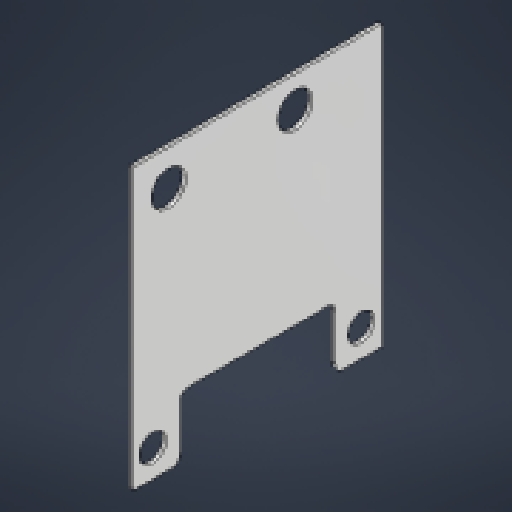
# Autodesk Inventor part: PLATE,FRONT
Saved by Autodesk Inventor 2026.1 (Build 301233020, 233B)
## iProperties
Created: 2026-03-30
Part Number: PLATE,FRONT
Material: Aluminum 6061-AHC
Document SubType Name: Sheet Metal
Designer: Owen L
Density: 2.7 g/cm^3
Sheet Metal Rule: Default
Appearance: Aluminum - Dark
Author: Owen L
Autodesk Inventor part; units mm, degrees
ref_plane "YZ Plane" through (0, 0, 0) normal (1, 0, 0) x (0, 1, 0)
ref_plane "XZ Plane" through (0, 0, 0) normal (0, 1, 0) x (-1, 0, 0)
ref_plane "XY Plane" through (0, 0, 0) normal (0, 0, 1) x (1, 0, 0)
sketch "Sketch1" plane through (0, 0, 0) normal (1, 0, 0) x (0, 1, 0)
  line L0 (-114.3, 101.6) -> (114.3, 101.6)
  line L1 (114.3, 101.6) -> (114.3, -101.6)
  line L2 (114.3, -101.6) -> (-114.3, -101.6)
  line L3 (-114.3, -101.6) -> (-114.3, 101.6)
  line L4 (-114.3, 101.6) -> (114.3, -101.6) construction
  line L5 (114.3, 101.6) -> (-114.3, -101.6) construction
  point P0 (0, 0)
  dimension "d0" = 228.6
  dimension "d1" = 203.2
  measures "d0" distance of L1.end L2.end
  measures "d1" distance of L0.end L1.end
extrude "Plate1" add sketch "Sketch1" along normal blind 3.175
sketch "Sketch2" plane through (3.175, 0, 0) normal (1, 0, 0) x (0, 0, -1)
  line L0 (-101.6, -114.3) -> (-101.6, 114.3) projected
  line L1 (-101.6, 114.3) -> (101.6, 114.3) projected
  circle A0 centre (-73.025, 85.217) radius 11.1125
  circle A1 centre (-85.725, -94.488) radius 11.1125
  circle A2 centre (84.455, -94.488) radius 11.1125
  line L2 (101.6, 114.3) -> (101.6, -114.3) projected
  circle A3 centre (30.3984, 88.9) radius 11.1125
  point P0 (0, 0)
  dimension "d3" = 28.575
  dimension "d4" = 29.083
  dimension "d5" = 22.225
  dimension "d9" = 15.875
  dimension "d11" = 22.225
  dimension "d19" = 103.489
  dimension "d20" = 25.4
  dimension "d21" = 170.18
  dimension "d23" = 208.788
  constraints: 4 centre point, 2 equal radius, 1 coincident, 1 horizontal alignment
  measures "d3" distance from line of L0 point (-73.025, 85.217)
  measures "d4" distance from line of L1 point (-73.025, 85.217)
  measures "d5" diameter of A0
  measures "d9" distance from line of L0 A1.centre
  measures "d11" diameter of A1
  measures "d19" distance of point (-73.025, 85.217) A3.centre
  measures "d20" distance from line of L1 A3.centre
  measures "d21" distance of A1.centre A2.centre
  measures "d23" distance from line of A1.centre L1
extrude "Cut1" cut sketch "Sketch2" against normal blind 3.175
sketch "Sketch3" plane through (3.175, 0, 0) normal (1, 0, 0) x (0, 0, -1)
  line L0 (-101.6, -114.3) -> (101.6, -114.3) projected
  line L1 (-63.5, -114.3) -> (63.5, -114.3)
  line L2 (63.5, -114.3) -> (63.5, -63.5)
  line L3 (63.5, -63.5) -> (-63.5, -63.5)
  line L4 (-63.5, -63.5) -> (-63.5, -114.3)
  point P0 (0, 0)
  point P1 (0, -63.5)
  point P2 (0, -114.3)
  dimension "d12" = 127
  dimension "d13" = 50.8
  constraints: 8 end point, 2 midpoint, 2 parallel, 1 horizontal, 1 perpendicular, 1 point on line, 1 vertical alignment
  measures "d12" distance of L3.end L2.end
  measures "d13" distance of L3.end L1.start
extrude "Cut2" cut sketch "Sketch3" against normal blind 3.175
fillet "Corner Round1" radius 6.35 4 edges at (1.5875, -114.3, 63.5) (1.5875, -63.5, 63.5) (1.5875, -114.3, -63.5) (1.5875, -63.5, -63.5)
equation "\"d6\" = Thickness"
equation "\"d14\" = Thickness"
equation "\"d2\" = Thickness"
equation "\"BendRadius\" = Thickness"
equation "\"BendReliefWidth\" = Thickness"
equation "\"BendReliefDepth\" = 0.5 * Thickness"
equation "\"CornerReliefSize\" = 4 * Thickness"
equation "\"MinimumRemnant\" = 2 * Thickness"
equation "\"TransitionRadius\" = BendRadius"
equation "\"JacobiRadiusSize\" = BendRadius"
equation "\"GapSize\" = Thickness"
equation "\"Thickness\" = 3.175"
body "Solid1"
